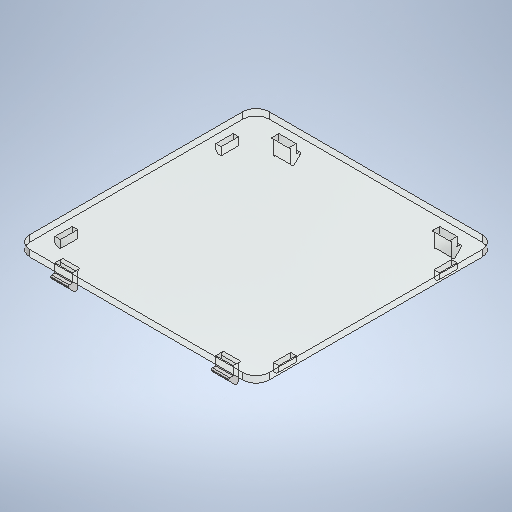
# Autodesk Inventor part: Cover side-2
Saved by Autodesk Inventor 2025 (Build 290162000, 162)
## iProperties
Created: 2025-08-11
Part Number: Cover side-2
Material: Generic
Document SubType Name: Modeling
Designer: yshis
Density: 1 g/cm^3
Appearance: Default
Author: yshis
Autodesk Inventor part; units mm, degrees
ref_plane "YZ Plane" through (0, 0, 0) normal (1, 0, 0) x (0, 1, 0)
ref_plane "XZ Plane" through (0, 0, 0) normal (0, 1, 0) x (-1, 0, 0)
ref_plane "XY Plane" through (0, 0, 0) normal (0, 0, 1) x (1, 0, 0)
sketch "Sketch1" plane through (0, 0, 0) normal (0, 1, 0) x (-1, 0, 0)
  line L0 (6, 0) -> (110, 0)
  line L1 (110, 0) -> (110, -104)
  line L2 (104, -110) -> (0, -110)
  line L3 (0, -110) -> (0, -6)
  arc A0 (104, -110) -> (110, -104) centre (104, -104) ccw
  arc A1 (6, 0) -> (0, -6) centre (6, -6) ccw
  point P0 (0, 0)
  point P1 (110, -110)
  dimension "d0" = 110
  dimension "d1" = 110
  dimension "d2" = 6
  constraints: 8 end point, 4 point on circle, 4 point on line, 4 tangent, 2 centre point, 2 parallel, 1 equal radius, 1 horizontal, 1 perpendicular
  measures "d0" distance of point (110, -110) L2.end
  measures "d1" distance of L0.end point (110, -110)
  measures "d2" radius of A0
extrude "Extrusion1" add sketch "Sketch1" along normal blind 3
fillet "Fillet1" radius 6 2 edges at (-110, 1.5, 0) (0, 1.5, -110)
sketch "Sketch3" plane through (0, 0, 0) normal (0, -1, 0) x (1, 0, 0)
  line L0 (-88, -106.5) -> (-96, -106.5)
  line L1 (-96, -106.5) -> (-96, -104)
  line L2 (-96, -104) -> (-88, -104)
  line L3 (-88, -104) -> (-88, -106.5)
  line L4 (-6, -110) -> (-104, -110) projected
  line L5 (-110, -104) -> (-110, -6) projected
  line L6 (-14, -106.5) -> (-22, -106.5)
  line L7 (-22, -106.5) -> (-22, -104)
  line L8 (-22, -104) -> (-14, -104)
  line L9 (-14, -104) -> (-14, -106.5)
  line L10 (-88, -6) -> (-96, -6)
  line L11 (-96, -6) -> (-96, -3.5)
  line L12 (-96, -3.5) -> (-88, -3.5)
  line L13 (-88, -3.5) -> (-88, -6)
  line L14 (-14, -6) -> (-22, -6)
  line L15 (-22, -6) -> (-22, -3.5)
  line L16 (-22, -3.5) -> (-14, -3.5)
  line L17 (-14, -3.5) -> (-14, -6)
  line L18 (-106.5, -96) -> (-104, -96)
  line L19 (-104, -96) -> (-104, -88)
  line L20 (-104, -88) -> (-106.5, -88)
  line L21 (-106.5, -88) -> (-106.5, -96)
  line L22 (-106.5, -22) -> (-104, -22)
  line L23 (-104, -14) -> (-106.5, -14)
  line L24 (-104, -22) -> (-104, -14)
  line L25 (-106.5, -14) -> (-106.5, -22)
  line L26 (-6, -96) -> (-3.5, -96)
  line L27 (-3.5, -88) -> (-6, -88)
  line L28 (-3.5, -96) -> (-3.5, -88)
  line L29 (-6, -88) -> (-6, -96)
  line L30 (-6, -22) -> (-3.5, -22)
  line L31 (-3.5, -14) -> (-6, -14)
  line L32 (-3.5, -22) -> (-3.5, -14)
  line L33 (-6, -14) -> (-6, -22)
  point P0 (0, 0)
  dimension "d20" = 8
  dimension "d21" = 2.5
  dimension "d22" = 3.5
  dimension "d23" = 14
  dimension "d26" = 74
  dimension "d29" = 100.5
  dimension "d55" = 8
  dimension "d56" = 2.5
  dimension "d57" = 14
  dimension "d60" = 74
  dimension "d63" = 100.5
  dimension "d66" = 3.5
  constraints: 64 end point, 4 horizontal, 4 parallel, 2 perpendicular, 2 vertical, 48 other
  measures "d20" distance of L1.end L2.end
  measures "d21" distance of L0.end L1.end
  measures "d22" distance between parallel lines of L4 L0
  measures "d23" distance between parallel lines of L5 L1
  measures "d26" distance of L0.start L6.start
  measures "d29" distance of L0.start L10.start
  measures "d55" distance of L18.end L19.end
  measures "d56" distance of L19.end L20.end
  measures "d57" distance between parallel lines of L4 L18
  measures "d60" distance of L18.end L22.end
  measures "d63" distance of L18.end L26.end
  measures "d66" distance between parallel lines of L5 L21
extrude "Extrusion3" add sketch "Sketch3" along normal blind 8.1
sketch "Sketch4" plane through (-88, 0, -106.5) normal (0, 0, -1) x (-1, 0, 0)
  line L0 (0, 0) -> (0, -8.1) projected
  line L1 (8, -8.1) -> (0, -8.1)
  line L2 (0, -8.1) -> (0, -4.1)
  line L3 (0, -4.1) -> (8, -4.1)
  line L4 (8, -4.1) -> (8, -8.1)
  line L5 (8, -8.1) -> (0, -8.1) projected
  line L6 (8, 0) -> (8, -8.1) projected
  line L7 (-66, 0) -> (-66, -8.1) projected
  line L8 (-74, 0) -> (-74, -8.1) projected
  line L9 (-66, -8.1) -> (-74, -8.1)
  line L10 (-74, -8.1) -> (-74, -4.1)
  line L11 (-74, -4.1) -> (-66, -4.1)
  line L12 (-66, -4.1) -> (-66, -8.1)
  point P0 (-88, 0)
  point P1 (0, -8.1)
  dimension "d34" = 4
  dimension "d35" = 0
  dimension "d36" = 0
  dimension "d37" = 4
  constraints: 16 end point, 4 parallel, 2 horizontal, 2 perpendicular, 2 point on line
  measures "d34" distance between parallel lines of L3 L1
  measures "d35" distance between parallel lines of L5 L1
  measures "d36" distance between parallel lines of L6 L4
  measures "d37" distance between parallel lines of L11 L9
extrude "Extrusion4" add sketch "Sketch4" along normal blind 2
chamfer "Chamfer1" distance 3 angle 45 2 edges at (-92, -8.1, -108.5) (-18, -8.1, -108.5)
fillet "Fillet2" radius 1 6 edges at (-92, -5.1, -108.5) (-18, -5.1, -108.5) (-18, -8.1, -105.5) (-92, -8.1, -105.5) (-92, -8.1, -104) (-18, -8.1, -104)
fillet "Fillet3" radius 0.5 2 edges at (-92, -4.1, -108.5) (-18, -4.1, -108.5)
sketch "Sketch5" plane through (-96, 0, -3.5) normal (0, 0, 1) x (1, 0, 0)
  line L0 (8, 0) -> (8, -8.1) projected
  line L1 (0, 0) -> (0, -8.1) projected
  line L2 (8, -8.1) -> (0, -8.1)
  line L3 (0, -8.1) -> (0, -4.05)
  line L4 (0, -4.05) -> (8, -4.05)
  line L5 (8, -4.05) -> (8, -8.1)
  line L6 (82, -8.1) -> (74, -8.1) projected
  line L7 (82, -8.1) -> (74, -8.1)
  line L8 (74, -8.1) -> (74, -4.1)
  line L9 (74, -4.1) -> (82, -4.1)
  line L10 (82, -4.1) -> (82, -8.1)
  point P0 (96, 0)
  point P1 (8, -4.05)
  dimension "d45" = 4.05
  constraints: 16 end point, 4 parallel, 2 horizontal, 2 perpendicular, 1 midpoint
  measures "d45" distance of L2.end L3.end
extrude "Extrusion5" add sketch "Sketch5" along normal blind 2
chamfer "Chamfer2" distance 3 angle 45 2 edges at (-92, -8.1, -1.5) (-18, -8.1, -1.5)
fillet "Fillet4" radius 1 6 edges at (-18, -8.1, -4.5) (-18, -5.1, -1.5) (-18, -8.1, -6) (-92, -8.1, -4.5) (-92, -5.1, -1.5) (-92, -8.1, -6)
fillet "Fillet5" radius 0.5 2 edges at (-92, -4.05, -1.5) (-18, -4.1, -1.5)
fillet "Fillet6" radius 1 1 edges at (-92, 0, -104)
fillet "Fillet7" radius 1 3 edges at (-18, 0, -104) (-18, 0, -6) (-92, 0, -6)
sketch "Sketch6" plane through (0, -8.1, 0) normal (0, -1, 0) x (1, 0, 0)
  line L0 (-104, -96) -> (-106.5, -96) projected
  line L1 (-104, -88) -> (-104, -96) projected
  line L2 (-106.5, -96) -> (-104, -96)
  line L3 (-104, -96) -> (-104, -88)
  line L4 (-104, -88) -> (-106.5, -88)
  line L5 (-106.5, -88) -> (-106.5, -96)
  line L6 (-106.5, -22) -> (-106.5, -14) projected
  line L7 (-106.5, -22) -> (-104, -22)
  line L8 (-104, -22) -> (-104, -14)
  line L9 (-104, -14) -> (-106.5, -14)
  line L10 (-106.5, -14) -> (-106.5, -22)
  line L11 (-6, -14) -> (-6, -22) projected
  line L12 (-3.5, -22) -> (-3.5, -14) projected
  line L13 (-6, -22) -> (-3.5, -22)
  line L14 (-3.5, -22) -> (-3.5, -14)
  line L15 (-3.5, -14) -> (-6, -14)
  line L16 (-6, -14) -> (-6, -22)
  line L17 (-3.5, -88) -> (-6, -88)
  line L18 (-6, -88) -> (-6, -96)
  line L19 (-6, -96) -> (-3.5, -96)
  line L20 (-3.5, -96) -> (-3.5, -88)
  point P0 (0, 0)
  constraints: 32 end point, 8 parallel, 5 point on line, 4 horizontal, 4 perpendicular
extrude "Extrusion6" cut sketch "Sketch6" against normal blind 4.5
chamfer "Chamfer3" distance 1 angle 45 4 edges at (-3.5, -3.6, -18) (-3.5, -3.6, -92) (-106.5, -3.6, -92) (-106.5, -3.6, -18)
equation "\"d26\" = d0 - d20 - 2 * d23"
equation "\"d29\" = d1 - d21 - 2 * d22"
equation "\"d55\" = d20"
equation "\"d56\" = d21"
equation "\"d57\" = d23"
equation "\"d60\" = d26"
equation "\"d63\" = d29"
equation "\"d66\" = d22"
body "Solid1"
